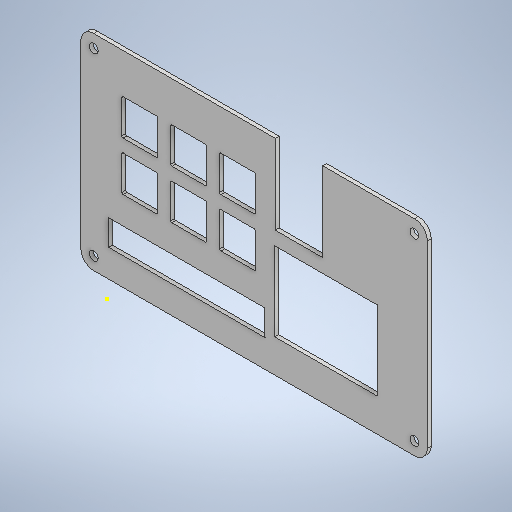
# Autodesk Inventor part: Top_Case
Saved by Autodesk Inventor 2025.1 (Build 291241000, 241)
## iProperties
Created: 2025-12-16
Part Number: Top_Case
Material: Generic
Document SubType Name: Modeling
Designer: omara
Density: 1 g/cm^3
Appearance: Default
Autodesk Inventor part; units mm, degrees
ref_plane "YZ Plane" through (0, 0, 0) normal (1, 0, 0) x (0, 1, 0)
ref_plane "XZ Plane" through (0, 0, 0) normal (0, 1, 0) x (-1, 0, 0)
ref_plane "XY Plane" through (0, 0, 0) normal (0, 0, 1) x (1, 0, 0)
sketch "Sketch1" plane through (0, 0, 0) normal (0, 0, 1) x (1, 0, 0)
  point P0 (0, 0)
sketch "0" plane through (0, 0, 0) normal (0, 0, 1) x (1, 0, 0)
  line L0 (7.6759, 72.8464) -> (20.6759, 72.8464)
  line L1 (7.6759, 58.8464) -> (20.6759, 58.8464)
  line L2 (7.1759, 72.3464) -> (7.1759, 59.3464)
  line L3 (21.1759, 72.3464) -> (21.1759, 59.3464)
  arc A0 (7.6759, 72.8464) -> (7.1759, 72.3464) centre (7.6759, 72.3464) ccw
  arc A1 (21.1759, 72.3464) -> (20.6759, 72.8464) centre (20.6759, 72.3464) ccw
  arc A2 (7.1759, 59.3464) -> (7.6759, 58.8464) centre (7.6759, 59.3464) ccw
  arc A3 (20.6759, 58.8464) -> (21.1759, 59.3464) centre (20.6759, 59.3464) ccw
  line L4 (26.7259, 72.8464) -> (39.7259, 72.8464)
  line L5 (26.7259, 58.8464) -> (39.7259, 58.8464)
  line L6 (26.2259, 72.3464) -> (26.2259, 59.3464)
  line L7 (40.2259, 72.3464) -> (40.2259, 59.3464)
  arc A4 (26.7259, 72.8464) -> (26.2259, 72.3464) centre (26.7259, 72.3464) ccw
  arc A5 (40.2259, 72.3464) -> (39.7259, 72.8464) centre (39.7259, 72.3464) ccw
  arc A6 (26.2259, 59.3464) -> (26.7259, 58.8464) centre (26.7259, 59.3464) ccw
  arc A7 (39.7259, 58.8464) -> (40.2259, 59.3464) centre (39.7259, 59.3464) ccw
  line L8 (45.7759, 72.8464) -> (58.7759, 72.8464)
  line L9 (45.7759, 58.8464) -> (58.7759, 58.8464)
  line L10 (45.2759, 72.3464) -> (45.2759, 59.3464)
  line L11 (59.2759, 72.3464) -> (59.2759, 59.3464)
  arc A8 (45.7759, 72.8464) -> (45.2759, 72.3464) centre (45.7759, 72.3464) ccw
  arc A9 (59.2759, 72.3464) -> (58.7759, 72.8464) centre (58.7759, 72.3464) ccw
  arc A10 (45.2759, 59.3464) -> (45.7759, 58.8464) centre (45.7759, 59.3464) ccw
  arc A11 (58.7759, 58.8464) -> (59.2759, 59.3464) centre (58.7759, 59.3464) ccw
  line L12 (7.6759, 53.7964) -> (20.6759, 53.7964)
  line L13 (7.6759, 39.7964) -> (20.6759, 39.7964)
  line L14 (7.1759, 53.2964) -> (7.1759, 40.2964)
  line L15 (21.1759, 53.2964) -> (21.1759, 40.2964)
  arc A12 (7.6759, 53.7964) -> (7.1759, 53.2964) centre (7.6759, 53.2964) ccw
  arc A13 (21.1759, 53.2964) -> (20.6759, 53.7964) centre (20.6759, 53.2964) ccw
  arc A14 (7.1759, 40.2964) -> (7.6759, 39.7964) centre (7.6759, 40.2964) ccw
  arc A15 (20.6759, 39.7964) -> (21.1759, 40.2964) centre (20.6759, 40.2964) ccw
  line L16 (26.7259, 53.7964) -> (39.7259, 53.7964)
  line L17 (26.7259, 39.7964) -> (39.7259, 39.7964)
  line L18 (26.2259, 53.2964) -> (26.2259, 40.2964)
  line L19 (40.2259, 53.2964) -> (40.2259, 40.2964)
  arc A16 (26.7259, 53.7964) -> (26.2259, 53.2964) centre (26.7259, 53.2964) ccw
  arc A17 (40.2259, 53.2964) -> (39.7259, 53.7964) centre (39.7259, 53.2964) ccw
  arc A18 (26.2259, 40.2964) -> (26.7259, 39.7964) centre (26.7259, 40.2964) ccw
  arc A19 (39.7259, 39.7964) -> (40.2259, 40.2964) centre (39.7259, 40.2964) ccw
  line L20 (45.7759, 53.7964) -> (58.7759, 53.7964)
  line L21 (45.7759, 39.7964) -> (58.7759, 39.7964)
  line L22 (45.2759, 53.2964) -> (45.2759, 40.2964)
  line L23 (59.2759, 53.2964) -> (59.2759, 40.2964)
  arc A20 (45.7759, 53.7964) -> (45.2759, 53.2964) centre (45.7759, 53.2964) ccw
  arc A21 (59.2759, 53.2964) -> (58.7759, 53.7964) centre (58.7759, 53.2964) ccw
  arc A22 (45.2759, 40.2964) -> (45.7759, 39.7964) centre (45.7759, 40.2964) ccw
  arc A23 (58.7759, 39.7964) -> (59.2759, 40.2964) centre (58.7759, 40.2964) ccw
  line L24 (-8.7991, 8.4184) -> (126.2009, 8.4184)
  line L25 (126.2009, 8.4184) -> (126.2009, 88.4184)
  line L26 (126.2009, 88.4184) -> (-8.7991, 88.4184)
  line L27 (-8.7991, 88.4184) -> (-8.7991, 8.4184)
  line L28 (66.9509, 88.4184) -> (85.4509, 88.4184)
  line L29 (85.4509, 88.4184) -> (85.4509, 57.4184)
  line L30 (85.4509, 57.4184) -> (66.9509, 57.4184)
  line L31 (66.9509, 57.4184) -> (66.9509, 88.4184)
  circle A24 centre (-3.7991, 83.4184) radius 1.7
  circle A25 centre (121.2009, 83.4184) radius 1.7
  circle A26 centre (121.2009, 13.4184) radius 1.7
  circle A27 centre (-3.7991, 13.4184) radius 1.7
  dimension "d2" = 135
  dimension "d3" = 80
  dimension "d4" = 15.975
  dimension "d5" = 15.572
  dimension "d6" = 18.5
  dimension "d7" = 31
  dimension "d8" = 75.75
  dimension "d9" = 3.4
  dimension "d10" = 3.4
  dimension "d11" = 3.4
  dimension "d12" = 3.4
  dimension "d13" = 5
  dimension "d14" = 5
  dimension "d15" = 5
  dimension "d16" = 5
  dimension "d17" = 5
  dimension "d18" = 5
  dimension "d19" = 5
  dimension "d20" = 5
  constraints: 64 end point, 48 point on circle, 28 centre point, 14 horizontal, 12 vertical, 4 perpendicular, 2 parallel, 1 point on line, 144 other
  measures "d2" distance of L24.start L24.end
  measures "d3" distance of L24.end L25.end
  measures "d4" distance between parallel lines of L2 L27
  measures "d5" distance between parallel lines of L0 L26
  measures "d6" distance of L29.end L30.end
  measures "d7" distance of L28.end L29.end
  measures "d8" distance between parallel lines of L27 L31
  measures "d9" diameter of A24
  measures "d10" diameter of A25
  measures "d11" diameter of A26
  measures "d12" diameter of A27
  measures "d13" distance from line of L26 A24.centre
  measures "d14" distance from line of L27 A24.centre
  measures "d15" distance from line of L24 A27.centre
  measures "d16" distance from line of L27 A27.centre
  measures "d17" distance from line of L25 A26.centre
  measures "d18" distance from line of L24 A26.centre
  measures "d19" distance from line of L25 A25.centre
  measures "d20" distance from line of L26 A25.centre
extrude "Extrusion1" add sketch "0" along normal blind 1.5 contours L27 L26 L31 L30 L29 L25 L24
sketch "Sketch4" plane through (0, 0, 1.5) normal (0, 0, 1) x (1, 0, 0)
  line L0 (0.7009, 78.9184) -> (116.7009, 78.9184)
  line L1 (116.7009, 78.9184) -> (116.7009, 17.9184)
  line L2 (116.7009, 17.9184) -> (0.7009, 17.9184)
  line L3 (0.7009, 17.9184) -> (0.7009, 78.9184)
  line L4 (66.9509, 88.4184) -> (-8.7991, 88.4184) projected
  line L5 (126.2009, 8.4184) -> (126.2009, 88.4184) projected
  line L6 (-8.7991, 8.4184) -> (126.2009, 8.4184) projected
  line L7 (-8.7991, 88.4184) -> (-8.7991, 8.4184) projected
  line L8 (66.7009, 52.0684) -> (106.7009, 52.0684)
  line L9 (106.7009, 52.0684) -> (106.7009, 21.3184)
  line L10 (106.7009, 21.3184) -> (66.7009, 21.3184)
  line L11 (66.7009, 21.3184) -> (66.7009, 52.0684)
  line L12 (85.4509, 57.4184) -> (66.9509, 57.4184) projected
  point P0 (0, 0)
  dimension "d23" = 9.5
  dimension "d24" = 9.5
  dimension "d25" = 9.5
  dimension "d26" = 9.5
  dimension "d27" = 5.35
  dimension "d28" = 30.75
  dimension "d29" = 40
  dimension "d30" = 10
  constraints: 16 end point, 4 parallel, 2 horizontal, 2 perpendicular
  measures "d23" distance between parallel lines of L4 L0
  measures "d24" distance between parallel lines of L5 L1
  measures "d25" distance between parallel lines of L6 L2
  measures "d26" distance between parallel lines of L7 L3
  measures "d27" distance between parallel lines of L8 L12
  measures "d28" distance between parallel lines of L10 L8
  measures "d29" distance between parallel lines of L9 L11
  measures "d30" distance between parallel lines of L1 L9
extrude "Extrusion2" cut sketch "Sketch4" against normal blind 1.5 contours L8 L9 L10 L11
sketch "Sketch5" plane through (0, 0, 1.5) normal (0, 0, 1) x (1, 0, 0)
  line L0 (1.9509, 29.1684) -> (62.9509, 29.1684)
  line L1 (62.9509, 29.1684) -> (62.9509, 19.1684)
  line L2 (62.9509, 19.1684) -> (1.9509, 19.1684)
  line L3 (1.9509, 19.1684) -> (1.9509, 29.1684)
  line L4 (-8.7991, 8.4184) -> (126.2009, 8.4184) projected
  line L5 (-8.7991, 88.4184) -> (-8.7991, 8.4184) projected
  point P0 (0, 0)
  dimension "d33" = 61
  dimension "d34" = 10
  dimension "d35" = 10.75
  dimension "d36" = 10.75
  constraints: 8 end point, 2 parallel, 1 horizontal, 1 perpendicular
  measures "d33" distance of L1.end L2.end
  measures "d34" distance of L0.end L1.end
  measures "d35" distance between parallel lines of L4 L2
  measures "d36" distance between parallel lines of L5 L3
extrude "Extrusion3" cut sketch "Sketch5" against normal blind 1.5
fillet "Fillet1" radius 5 4 edges at (-8.7991, 8.4184, 0.75) (-8.7991, 88.4184, 0.75) (126.2009, 88.4184, 0.75) (126.2009, 8.4184, 0.75)
body "Solid1"
